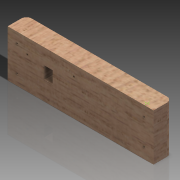
# Autodesk Inventor part: Seitenteil_mit_schalter
Saved by Autodesk Inventor 2014 SP1 (Build 180222100, 222)
## iProperties
Created: 2017-12-30
Part Number: Seitenteil_mit_schalter
Material: Eiche, weiß
Document SubType Name: Modeling
Designer: Flo
Density: 0.721 g/cm^3
Appearance: Weißeiche - massiv - natur - mittlerer Glanz
Mass: 79.7838 g
Surface Area: 201.786 cm^2
Volume: 110.657 cm^3
Author: Flo
Autodesk Inventor part; units mm, degrees
ref_plane "YZ Plane" through (0, 0, 0) normal (1, 0, 0) x (0, 1, 0)
ref_plane "XZ Plane" through (0, 0, 0) normal (0, 1, 0) x (-1, 0, 0)
ref_plane "XY Plane" through (0, 0, 0) normal (0, 0, 1) x (1, 0, 0)
sketch "Skizze1" plane through (0, 0, 0) normal (0, 1, 0) x (-1, 0, 0)
  line L0 (0, 0) -> (140, 0)
  line L1 (140, 0) -> (140, -45)
  line L2 (140, -45) -> (0, -45)
  line L3 (0, -45) -> (0, 0)
  dimension "d0" = 140
  dimension "d1" = 45
  constraints: 8 end point, 2 parallel, 1 horizontal, 1 perpendicular
  measures "d0" distance of L1.end L2.end
  measures "d1" distance of L0.end L1.end
extrude "Extrusion1" add sketch "Skizze1" along normal blind 18
sketch "Skizze2" plane through (0, 18, 0) normal (0, 1, 0) x (1, 0, 0)
  line L0 (0, 0) -> (0, 45) projected
  line L1 (0, 45) -> (-140, 45) projected
  line L2 (-140, 45) -> (-140, 0) projected
  point P0 (-131, 35)
  point P1 (-131, 10)
  point P2 (-9, 35)
  point P3 (-9, 10)
  dimension "d14" = 10
  dimension "d15" = 25
  dimension "d16" = 10
  dimension "d17" = 25
  dimension "d18" = 9
  dimension "d19" = 9
  measures "d14" distance from line of L1 point (-131, 35)
  measures "d15" distance of point (-131, 10) point (-131, 35)
  measures "d16" distance from line of L1 point (-9, 35)
  measures "d17" distance of point (-9, 35) point (-9, 10)
  measures "d18" distance from line of L0 point (-9, 35)
  measures "d19" distance from line of L2 point (-131, 35)
hole "Bohrung1" at (-131, 18, -35) at (-131, 18, -10) at (-9, 18, -35) at (-9, 18, -10) direction (0, -1, 0) diameter 2 end through all countersink diameter 5 countersink angle 90
fillet "Rundung3" radius 5 2 edges at (0, 18, -22.5) (-140, 18, -22.5)
sketch "Skizze3" plane through (0, 18, 0) normal (0, 1, 0) x (1, 0, 0)
  line L0 (-135, 0) -> (-5, 0) projected
  line L1 (-97, 15) -> (-105, 15)
  line L2 (-105, 15) -> (-105, 27)
  line L3 (-105, 27) -> (-97, 27)
  line L4 (-97, 27) -> (-97, 15)
  line L5 (0, 0) -> (0, 45) projected
  line L6 (-140, 45) -> (-140, 0) projected
  dimension "d32" = 8
  dimension "d33" = 12
  dimension "d34" = 15
  dimension "d36" = 35
  constraints: 8 end point, 2 parallel, 1 horizontal, 1 perpendicular
  measures "d32" distance of L2.end L3.end
  measures "d33" distance of L3.end L1.start
  measures "d34" distance between parallel lines of L0 L1
  measures "d36" distance between parallel lines of L6 L2
extrude "Extrusion2" cut sketch "Skizze3" against normal blind 18
sketch "Skizze4" plane through (-140, 0, 0) normal (0, 0, 1) x (1, 0, 0)
  point P0 (131, 3)
